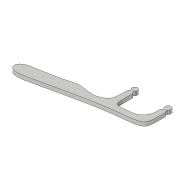
# Autodesk Inventor part: toothpick
Saved by Autodesk Inventor 2019.4 (Build 234330000, 330)
## iProperties
Created: 2021-03-17
Part Number: toothpick
Material: Generic
Document SubType Name: Modeling
Designer: diederichbenedict
Density: 1 g/cm^3
Appearance: Default
Author: diederichbenedict
Autodesk Inventor part; units mm, degrees
ref_plane "YZ Plane" through (0, 0, 0) normal (1, 0, 0) x (0, 1, 0)
ref_plane "XZ Plane" through (0, 0, 0) normal (0, 1, 0) x (-1, 0, 0)
ref_plane "XY Plane" through (0, 0, 0) normal (0, 0, 1) x (1, 0, 0)
sketch "Sketch1" plane through (0, 0, 0) normal (0, 1, 0) x (-1, 0, 0)
  line L0 (0, 0) -> (228.0708, 0) construction
  line L1 (228.0708, 0) -> (228.0708, -146.5792) construction
  line L2 (228.0708, -146.5792) -> (0, -146.5792) construction
  line L3 (0, -146.5792) -> (0, 0) construction
  line L4 (102.5046, -125.6494) -> (92.2803, -127.3628) construction
  line L5 (92.2803, -127.3628) -> (88.4939, -128.901) construction
  line L6 (88.4939, -128.901) -> (86.8374, -128.901) construction
  line L7 (86.8374, -128.901) -> (82.9327, -128.2206) construction
  line L8 (82.9327, -128.2206) -> (80.2704, -128.0432) construction
  line L9 (80.2704, -128.0432) -> (77.6081, -129.2264) construction
  line L10 (77.6081, -129.2264) -> (76.4545, -130.2321) construction
  line L11 (76.4545, -130.2321) -> (75.715, -132.0957) construction
  line L12 (75.715, -132.0957) -> (75.8924, -137.8936) construction
  line L13 (75.8924, -137.8936) -> (75.8924, -139.0177) construction
  line L14 (75.8924, -139.0177) -> (74.7092, -139.5501) construction
  line L15 (74.7092, -139.5501) -> (73.7035, -139.0472) construction
  line L16 (73.7035, -139.0472) -> (73.7035, -137.8048) construction
  line L17 (73.7035, -137.8048) -> (73.7035, -131.1492) construction
  line L18 (73.7035, -131.1492) -> (73.4964, -129.1081) construction
  line L19 (73.4964, -129.1081) -> (71.899, -129.2856) construction
  line L20 (71.899, -129.2856) -> (65.1546, -129.818) construction
  line L21 (65.1546, -129.818) -> (62.9254, -130.5302) construction
  spline S0 degree 4 poles (102.5046, -125.6494) (92.2803, -127.3628) (88.4939, -128.901) (86.8374, -128.901) (82.9327, -128.2206) (80.2704, -128.0432) (77.6081, -129.2264) (76.4545, -130.2321) (75.715, -132.0957) (75.8924, -137.8936) (75.8924, -139.0177) (74.7092, -139.5501) (73.7035, -139.0472) (73.7035, -137.8048) (73.7035, -131.1492) (73.4964, -129.1081) (71.899, -129.2856) (65.1546, -129.818) (62.9254, -130.5302) knots 1 1 1 1 1 2 3 4 5 6 7 8 9 10 11 12 13 14 15 16 16 16 16 16
  line L22 (62.9254, -130.5302) -> (62.9254, -137.538) construction
  line L23 (62.9254, -137.538) -> (62.83, -138.9678) construction
  line L24 (62.83, -138.9678) -> (62.7627, -139.3543) construction
  line L25 (62.7627, -139.3543) -> (61.7519, -139.5937) construction
  line L26 (61.7519, -139.5937) -> (60.7033, -139.359) construction
  line L27 (60.7033, -139.359) -> (60.7736, -138.9557) construction
  line L28 (60.7736, -138.9557) -> (60.7736, -130.7036) construction
  line L29 (60.7736, -130.7036) -> (61.0687, -127.9988) construction
  line L30 (61.0687, -127.9988) -> (68.63, -127.2994) construction
  line L31 (68.63, -127.2994) -> (76.3781, -126.596) construction
  line L32 (76.3781, -126.596) -> (99.3029, -121.4351) construction
  line L33 (99.3029, -121.4351) -> (104.5008, -120.204) construction
  line L34 (104.5008, -120.204) -> (107.4559, -121.6816) construction
  line L35 (107.4559, -121.6816) -> (106.9842, -124.3889) construction
  line L36 (106.9842, -124.3889) -> (104.0673, -125.3875) construction
  line L37 (104.0673, -125.3875) -> (102.5046, -125.6494) construction
  spline S1 degree 4 poles (62.9254, -130.5302) (62.9254, -137.538) (62.83, -138.9678) (62.7627, -139.3543) (61.7519, -139.5937) (60.7033, -139.359) (60.7736, -138.9557) (60.7736, -130.7036) (61.0687, -127.9988) (68.63, -127.2994) (76.3781, -126.596) (99.3029, -121.4351) (104.5008, -120.204) (107.4559, -121.6816) (106.9842, -124.3889) (104.0673, -125.3875) (102.5046, -125.6494) knots 1 1 1 1 1 2 3 4 5 6 7 8 9 10 11 12 13 14 14 14 14 14
  constraints: 5 vertical, 1 horizontal, 8 other
extrude "Extrusion1" add sketch "Sketch1" along normal blind 1.5
fillet "Fillet1" radius 5 1 edges at (-62.9254, 0.75, -130.5302)
sketch "Sketch2" plane through (0, 1.5, 0) normal (0, 1, 0) x (1, 0, 0)
  circle A0 centre (-75.8584, 137.1775) radius 0.5167
  circle A1 centre (-73.7098, 137.1775) radius 0.5292
  circle A2 centre (-62.8907, 137.1775) radius 0.519
  circle A3 centre (-60.7639, 137.1775) radius 0.5274
  point P0 (0, 0)
  constraints: 4 centre point, 7 other
extrude "Extrusion2" cut sketch "Sketch2" against normal through all
fillet "Fillet2" radius 0.5 8 edges at (-73.7209, 0.75, -137.7066) (-73.7051, 0.75, -136.6483) (-75.8515, 0.75, -136.6609) (-75.859, 0.75, -137.6942) (-62.8991, 0.75, -136.6586) (-62.8787, 0.75, -137.6964) (-60.7671, 0.75, -136.6502) (-60.762, 0.75, -137.7049)
body "Solid1"
